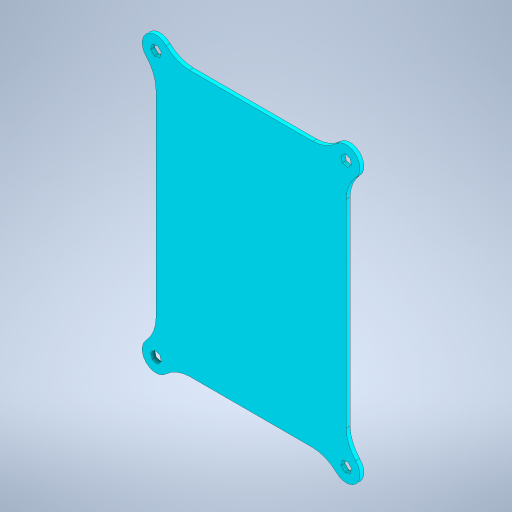
# Autodesk Inventor part: TUTUP
Saved by Autodesk Inventor 2024 (Build 280153000, 153)
## iProperties
Created: 2024-10-13
Part Number: TUTUP
Material: Generic
Document SubType Name: Modeling
Designer: Lenovo
Density: 1 g/cm^3
Appearance: Default
Author: Lenovo
Autodesk Inventor part; units mm, degrees
ref_plane "YZ Plane" through (0, 0, 0) normal (1, 0, 0) x (0, 1, 0)
ref_plane "XZ Plane" through (0, 0, 0) normal (0, 1, 0) x (-1, 0, 0)
ref_plane "XY Plane" through (0, 0, 0) normal (0, 0, 1) x (1, 0, 0)
sketch "Sketch1" plane through (0, 0, 0) normal (0, 0, 1) x (1, 0, 0)
  line L0 (-43.5, 62.5) -> (43.5, 62.5)
  line L1 (43.5, 62.5) -> (43.5, -62.7974)
  line L2 (43.5, -62.7974) -> (-43.5, -62.7974)
  line L3 (-43.5, -62.5) -> (-43.5, 62.5)
  line L4 (-43.5, 62.5) -> (43.5, -62.7974) construction
  line L5 (43.5, 62.5) -> (-43.5, -62.7974) construction
  line L6 (-53.5, 72.3513) -> (53.5, -72.6487) construction
  line L7 (53.5, 72.3513) -> (-53.5, -72.6487) construction
  line L8 (-46.5555, 65.5555) -> (-49.2118, 64.8437)
  line L9 (-49.2118, 64.8437) -> (-51.1563, 66.7882)
  line L10 (-51.1563, 66.7882) -> (-50.4445, 69.4445)
  line L11 (-50.4445, 69.4445) -> (-47.7882, 70.1563)
  line L12 (-47.7882, 70.1563) -> (-45.8437, 68.2118)
  line L13 (-45.8437, 68.2118) -> (-46.5555, 65.5555)
  line L14 (-43.5, 62.5) -> (43.5, 62.5)
  line L15 (-43.5, 62.5) -> (-43.5, -62.7974)
  line L16 (-31.4289, 67.5) -> (31.4289, 67.5)
  line L17 (-48.5, -50.7264) -> (-48.5, 50.4289)
  arc A0 (-48.5, 50.4289) -> (-53.3593, 62.3516) centre (-66.4959, 50.0459) ccw
  arc A1 (-43.3524, 72.3601) -> (-31.4289, 67.5) centre (-31.0458, 85.4959) ccw
  arc A2 (-43.3524, 72.3601) -> (-53.3593, 62.3516) centre (-48.5, 67.5) ccw
  arc A3 (53.3593, 62.3516) -> (48.5, 50.4289) centre (66.4959, 50.0459) ccw
  arc A4 (31.4289, 67.5) -> (43.3524, 72.3601) centre (31.0458, 85.4959) ccw
  line L18 (53.5, 72.3513) -> (-53.5, -72.6487) construction
  line L19 (46.5555, 65.5555) -> (49.2118, 64.8437)
  line L20 (51.1563, 66.7882) -> (50.4445, 69.4445)
  line L21 (50.4445, 69.4445) -> (47.7882, 70.1563)
  line L22 (47.7882, 70.1563) -> (45.8437, 68.2118)
  arc A5 (53.3593, 62.3516) -> (43.3524, 72.3601) centre (48.5, 67.5) ccw
  line L23 (49.2118, 64.8437) -> (51.1563, 66.7882)
  line L24 (45.8437, 68.2118) -> (46.5555, 65.5555)
  line L25 (48.5, -50.7264) -> (48.5, 50.4289)
  line L26 (53.5, -72.6487) -> (-53.5, 72.3513) construction
  line L27 (53.5, -72.6487) -> (-53.5, 72.3513) construction
  line L28 (-53.5, -72.6487) -> (53.5, 72.3513) construction
  line L29 (-46.5555, -65.8529) -> (-49.2118, -65.1411)
  line L30 (-45.8437, -68.5092) -> (-46.5555, -65.8529)
  line L31 (-49.2118, -65.1411) -> (-51.1563, -67.0857)
  line L32 (-47.7882, -70.4537) -> (-45.8437, -68.5092)
  line L33 (-51.1563, -67.0857) -> (-50.4445, -69.742)
  line L34 (-50.4445, -69.742) -> (-47.7882, -70.4537)
  line L35 (45.8437, -68.5092) -> (46.5555, -65.8529)
  line L36 (47.7882, -70.4537) -> (45.8437, -68.5092)
  line L37 (46.5555, -65.8529) -> (49.2118, -65.1411)
  line L38 (50.4445, -69.742) -> (47.7882, -70.4537)
  line L39 (51.1563, -67.0857) -> (50.4445, -69.742)
  line L40 (49.2118, -65.1411) -> (51.1563, -67.0857)
  arc A6 (43.3524, -72.6576) -> (31.4289, -67.7974) centre (31.0458, -85.7934) ccw
  arc A7 (43.3524, -72.6576) -> (53.3593, -62.6491) centre (48.5, -67.7974) ccw
  arc A8 (-31.4289, -67.7974) -> (-43.3524, -72.6576) centre (-31.0458, -85.7934) ccw
  arc A9 (-53.3593, -62.6491) -> (-43.3524, -72.6576) centre (-48.5, -67.7974) ccw
  arc A10 (-53.3593, -62.6491) -> (-48.5, -50.7264) centre (-66.4959, -50.3434) ccw
  arc A11 (48.5, -50.7264) -> (53.3593, -62.6491) centre (66.4959, -50.3434) ccw
  line L41 (-31.4289, -67.7974) -> (31.4289, -67.7974)
  point P0 (0, 0)
  point P1 (-3.5, -17.5)
  dimension "d0" = 87
  dimension "d1" = 107
  dimension "d2" = 145
  dimension "d4" = 5
  dimension "d5" = 5
  constraints: 84 end point, 24 point on circle, 12 centre point, 4 coincident, 4 parallel, 2 perpendicular, 1 collinear, 1 horizontal, 13 other
  measures "d0" distance of L2.end L2.start
  measures "d1" distance of L6.end L7.end
  measures "d2" distance of L7.start L6.end
  measures "d4" distance between parallel lines of L0 L16
  measures "d5" distance between parallel lines of L3 L17
extrude "Extrusion1" add sketch "Sketch1" against normal blind 2
extrude "Extrusion2" add sketch "Sketch1" against normal blind 5 contours L0 L1 L2 L15 L3
body "Solid1"
